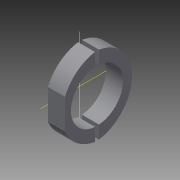
# Autodesk Inventor part: turny_bit
Saved by Autodesk Inventor 2015 (Build 190159000, 159)
## iProperties
Created: 2015-09-23
Part Number: turny_bit
Material: Generic
Description: insert part description/title
Document SubType Name: Modeling
Designer: francis
Density: 1 g/cm^3
Appearance: Default
Author: francis
Part Category: insert part category here and press enter to fill value
Autodesk Inventor part; units mm, degrees
ref_plane "YZ Plane" through (0, 0, 0) normal (1, 0, 0) x (0, 1, 0)
ref_plane "XZ Plane" through (0, 0, 0) normal (0, 1, 0) x (-1, 0, 0)
ref_plane "XY Plane" through (0, 0, 0) normal (0, 0, 1) x (1, 0, 0)
sketch "Sketch1" plane through (0, 0, 0) normal (1, 0, 0) x (0, 1, 0)
  arc A0 (2, -38.923) -> (2, 38.923) centre (-4.4545, 0) ccw
  line L0 (0, -54.4921) -> (0, 54.4921) construction
  line L1 (2, 38.923) -> (2, 25.923)
  line L2 (2, -38.923) -> (2, -25.923)
  line L3 (-49, 0) -> (49, 0) construction
  arc A1 (2, -25.923) -> (2, 25.923) centre (0, 0) ccw
  arc A2 (-2, 38.923) -> (-2, -38.923) centre (4.4545, 0) ccw
  line L4 (-2, 38.923) -> (-2, 25.923)
  line L5 (-2, -38.923) -> (-2, -25.923)
  arc A3 (-2, 25.923) -> (-2, -25.923) centre (0, 0) ccw
  point P0 (0, 0)
  point P1 (12.8231, 0)
  point P2 (35, 0)
  point P3 (12.8231, 0)
  point P4 (26, 0)
  point P5 (-12.8231, 0)
  point P6 (-35, 0)
  point P7 (-12.8231, 0)
  point P8 (-26, 0)
  dimension "d2" = 13
  dimension "d6" = 26
  dimension "d7" = 9
  dimension "d9" = 33
  constraints: 10 point on circle, 9 symmetric about line, 8 end point, 4 centre point, 2 coincident, 2 collinear, 2 point on line, 1 midpoint, 1 vertical, 3 other
  measures "d2" distance of L1.start L1.end
  measures "d6" radius of A1
  measures "d7" distance of point (26, 0) point (35, 0)
  measures "d9" distance from line of L1 point (35, 0)
extrude "Extrusion1" add sketch "Sketch1" along normal blind 17
sketch "Sketch5" plane through (17, 0, 0) normal (1, 0, 0) x (0, 0, -1)
  line L0 (38.923, -2) -> (25.923, -2) construction
  arc A0 (-25.923, -2) -> (25.923, -2) centre (0, 0) ccw construction
  line L1 (-25.923, -2) -> (-38.923, -2) construction
  arc A1 (-38.923, -2) -> (38.923, -2) centre (0, 4.4545) ccw construction
  line L2 (0, -49) -> (0, 49) construction
  arc A2 (-25.923, -2) -> (25.923, -2) centre (0, 0) ccw construction
  line L3 (15.0906, -35) -> (-15.0906, -35)
  line L4 (-15.0906, -35) -> (-15.0906, -32)
  line L5 (-15.0906, -32) -> (15.0906, -32)
  line L6 (15.0906, -32) -> (15.0906, -35)
  arc A3 (-38.923, -2) -> (38.923, -2) centre (0, 4.4545) ccw projected
  point P0 (0, 0)
  point P1 (0, -26)
  dimension "d13" = 6
  constraints: 8 end point, 3 point on circle, 2 parallel, 1 horizontal, 1 perpendicular, 1 point on line, 1 tangent
  measures "d13" distance from line of L5 point (0, -26)
extrude "Extrusion2" cut sketch "Sketch5" against normal blind 17
body "Solid1"
